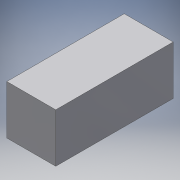
# Autodesk Inventor part: mockPi
Saved by Autodesk Inventor 2018 (Build 220112000, 112)
## iProperties
Created: 2020-10-03
Part Number: mockPi
Material: Generic
Document SubType Name: Modeling
Designer: Lveli
Density: 1 g/cm^3
Appearance: White
Author: Lveli
Autodesk Inventor part; units mm, degrees
ref_plane "YZ Plane" through (0, 0, 0) normal (1, 0, 0) x (0, 1, 0)
ref_plane "XZ Plane" through (0, 0, 0) normal (0, 1, 0) x (-1, 0, 0)
ref_plane "XY Plane" through (0, 0, 0) normal (0, 0, 1) x (1, 0, 0)
sketch "Sketch1" plane through (0, 0, 0) normal (0, 1, 0) x (-1, 0, 0)
  line L0 (-15.875, 38.1) -> (15.875, 38.1)
  line L1 (15.875, 38.1) -> (15.875, -38.1)
  line L2 (15.875, -38.1) -> (-15.875, -38.1)
  line L3 (-15.875, -38.1) -> (-15.875, 38.1)
  line L4 (-15.875, 38.1) -> (15.875, -38.1) construction
  line L5 (15.875, 38.1) -> (-15.875, -38.1) construction
  point P0 (0, 0)
  dimension "d0" = 76.2
  dimension "d1" = 31.75
  constraints: 12 end point, 2 midpoint, 2 parallel, 1 horizontal, 1 perpendicular
  measures "d0" distance of L0.end L1.end
  measures "d1" distance of L0.start L0.end
extrude "Extrusion1" add sketch "Sketch1" along normal blind 31.75
body "Solid1"
